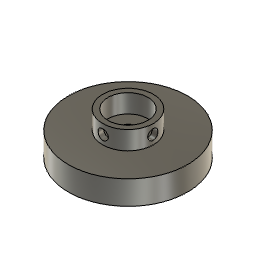
Tool change - tool mount three magnets (Autodesk Fusion 360 design; units mm, degrees)
Autodesk Fusion 360 part; units mm, degrees
note: some values were not read from the file. Set by a fixed rule: which face or edge a step refers to.
sketch "Sketch1" plane through (0, 0, 0) normal (0, 0, 1) x (1, 0, 0)
  circle A0 centre (0, 0) radius 20
  circle A1 centre (0, -12) radius 3.55
  circle A2 centre (0, 12) radius 3.55
  circle A3 centre (10.3923, -6) radius 3.55
  circle A4 centre (-10.3923, 6) radius 3.55
  circle A5 centre (-10.3923, -6) radius 3.55
  circle A6 centre (0, 0) radius 2.1
  line L0 (0, 0) -> (0, 12) construction
  line L1 (0, 0) -> (10.3923, -6) construction
  line L2 (0, 0) -> (10.3923, 6) construction
  circle A7 centre (10.3923, 6) radius 3.55
  dimension "d1" = 40
  dimension "d2" = 7.1
  dimension "d3" = 7.1
  dimension "d6" = 7.1
  dimension "d12" = 12
  dimension "d15" = 12
  dimension "d16" = 7.1
  dimension "d17" = 12
  dimension "d19" = 7.1
  dimension "d23" = 12
  dimension "d25" = 4.2
  dimension "d34" = 60
  dimension "d37" = 60
  dimension "d38" = 60
  dimension "d39" = 60
  dimension "d49" = 12
  dimension "d50" = 7.1
  dimension "d51" = 60
  dimension "d52" = 60
  dimension "d85" = 12
  constraint coincident A0.centre A6.centre
  constraint coincident A2.centre L0.end
  constraint vertical L0
  constraint coincident A3.centre L1.end
  constraint coincident L2.end A7.centre
  measures "d1" diameter of A0
  measures "d2" diameter of A1
  measures "d3" diameter of A2
  measures "d6" diameter of A3
  measures "d12" distance of A0.centre A2.centre
  measures "d15" distance of A0.centre A3.centre
  measures "d16" diameter of A4
  measures "d17" distance of A0.centre A4.centre
  measures "d19" diameter of A5
  measures "d23" distance of A0.centre A1.centre
  measures "d25" diameter of A6
  measures "d34" angle of A0.centre A1.centre A3.centre
  measures "d37" angle of A0.centre A2.centre A4.centre
  measures "d38" angle of A0.centre A4.centre A5.centre
  measures "d39" angle of A0.centre A1.centre A5.centre
  measures "d49" distance of A0.centre L2.end
  measures "d50" diameter of A7
  measures "d51" angle of L0 L2
  measures "d52" angle of L1 L2
  measures "d85" distance of A5.centre A0.centre
sketch "Sketch2" plane through (0, 0, 0) normal (0, 0, 1) x (1, 0, 0)
  circle A0 centre (0, 0) radius 20
  line L0 (0, 0) -> (0, -9) construction
  line L1 (0, 0) -> (0, 9) construction
  line L2 (20, -0.0372) -> (-20, -0.0372) construction
  line L3 (-14, -0.0372) -> (-20, -0.0372) construction
  dimension "d26" = 40
  dimension "d40" = 6
  constraint coincident A0.centre L0.start
  constraint coincident A0 L2.start
  constraint coincident A0 L2.end
  constraint horizontal L2
  constraint parallel L2 L3
  measures "d26" diameter of A0
  measures "d40" distance of L2.end L3.start
extrude "Extrude1" add sketch "Sketch2" along normal blind 5 and the other way blind 3
sketch "Sketch3" plane through (0, 0, 0) normal (0, 0, 1) x (1, 0, 0)
hole "Hole1" at (-0.003, -0.037, -3) direction (0, 0, 1) diameter 5.029 depth 14 tip angle 180 counterbore diameter 9 counterbore depth 5.4
thread "Thread1" "ISO Metric profile 5.5 M5.5x0.5 6H"
extrude "Extrude2" cut sketch "Sketch1" along normal blind -3 and the other way blind -0.2 contours A1 | A2 | A3 | A4 | A5
extrude "Extrude4" cut sketch "Sketch1" along normal blind 0.2 and the other way blind 3 contours A7
sketch "Sketch4" plane through (0, 0, 5) normal (0, 0, 1) x (-1, 0, 0)
  circle A0 centre (0.003, 0.037) radius 2.5143
  circle A1 centre (0, 0) radius 20
  circle A2 centre (0, 0) radius 6.5
  circle A3 centre (0, 0) radius 3
  dimension "d57" = 13
  dimension "d58" = 6
  constraint concentric A1 A2
  constraint concentric A2 A3
  measures "d57" diameter of A2
  measures "d58" diameter of A3
sketch "Sketch5" plane through (0, 0, 5) normal (0, 0, 1) x (-1, 0, 0)
  circle A0 centre (0, 0) radius 20
  circle A1 centre (0, 0) radius 8.5
  circle A2 centre (0, 0) radius 6.7
  circle A3 centre (0.003, 0.037) radius 2.5143
  dimension "d61" = 17
  dimension "d62" = 13.4
  constraint concentric A0 A1
  constraint concentric A1 A2
  measures "d61" diameter of A1
  measures "d62" diameter of A2
extrude "Extrude6" add sketch "Sketch5" along normal blind 6.2 contours A1
sketch "Sketch6" plane through (0, 0, 5) normal (0, 0, 1) x (-1, 0, 0)
  circle A0 centre (0, 0) radius 20
  circle A1 centre (0, 0) radius 8.5
  circle A2 centre (0, 0) radius 6.5
  dimension "d65" = 13
  constraint coincident A0.centre A1.centre
  measures "d65" diameter of A2
sketch "Sketch7" plane through (0, 0, 0) normal (1, 0, 0) x (0, 1, 0)
sketch "Sketch8" plane through (0, 0, 11.2) normal (0, 0, 1) x (-1, 0, 0)
  circle A0 centre (0, 0) radius 6.7
  circle A1 centre (0, 0) radius 8.5
sketch "Sketch9" plane through (0, 0, 11.2) normal (0, 0, 1) x (-1, 0, 0)
  line L0 (0, -8.4831) -> (0, 8.4366) construction
  line L1 (8.5, -0.0044) -> (-8.5, -0.0044) construction
  circle A0 centre (0, 0) radius 8.5 construction
  arc A1 (0, -8.4831) -> (6.3875, -5.608) centre (0.0534, -0.0686) ccw
  constraint vertical L0
  constraint horizontal L1
  constraint coincident L1.end A0
  constraint coincident L1.start A0
  constraint coincident A0 A1.end
extrude "Extrude3" cut sketch "Sketch1" along normal blind 3.2 contours A1 | A2 | A3 | A4 | A5 | A7
sketch "Sketch10" plane through (0, 0, 0) normal (1, 0, 0) x (0, 1, 0)
  circle A0 centre (0.01, 9) radius 1.5
  line L0 (0, 1.9) -> (0, 14.3)
  circle A1 centre (0.01, 9) radius 1.25
  dimension "d66" = 3
  dimension "d67" = 0.01
  dimension "d68" = 2.5
  constraint concentric A0 A1
  measures "d66" diameter of A0
  measures "d67" distance of A0.centre L0
  measures "d68" diameter of A1
sketch "Sketch11" plane through (0, 0, 0) normal (0, 1, 0) x (1, 0, 0)
  line L0 (0, -5) -> (0, -11) construction
  line L1 (0, -5) -> (0, -11) construction
  line L2 (0, -5) -> (0, -8) construction
  circle A0 centre (0, -8) radius 1.25
  circle A1 centre (0, -8) radius 1.7
  dimension "d69" = 3
  dimension "d70" = 2.5
  dimension "d86" = 3.4
  constraint vertical L0
  constraint parallel L1 L2
  constraint coincident L2.end A0.centre
  constraint concentric A0 A1
  measures "d69" distance of L0.start L2.end
  measures "d70" diameter of A0
  measures "d86" diameter of A1
extrude "Extrude7" cut sketch "Sketch11" against normal blind 19 contours A0
sketch "Sketch12" plane through (0, 0, 0) normal (1, 0, 0) x (0, 1, 0)
  line L0 (0, 5) -> (0, 11)
  line L1 (0, 11) -> (0, 8)
  circle A0 centre (0, 8) radius 1.25
  circle A1 centre (0, 8) radius 1.7
  dimension "d73" = 3
  dimension "d74" = 2.5
  dimension "d89" = 3.4
  constraint vertical L0
  constraint parallel L0 L1
  constraint coincident L1.end A0.centre
  constraint concentric A0 A1
  measures "d73" distance of L0.end L1.end
  measures "d74" diameter of A0
  measures "d89" diameter of A1
extrude "Extrude8" cut sketch "Sketch12" along normal blind 18 contours L0 L1 A0 | L0 L1 A0
extrude "Extrude9" cut sketch "Sketch11" against normal blind 11
extrude "Extrude10" cut sketch "Sketch12" along normal blind 15 contours L0 L1 A0 A1 | L0 L1 A0 A1
extrude "Extrude11" add 3 faces at (-10.4048, -6.9337, 3.2) (-0.8737, 12.0232, 3.2) (9.1513, -4.7203, 3.2) along direction (0, 0, -1) blind 6.2
extrude "Extrude12" add 3 faces at (-0.8737, -11.9768, 3.2) (9.7613, 6.2168, 3.2) (-11.4191, 6.8816, 3.2) along direction (0, 0, -1) blind 3
thread "Thread3" [suppressed]
